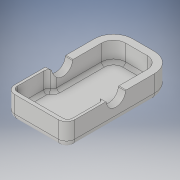
# Autodesk Inventor part: Component 27 (Bracket Cover)
Saved by Autodesk Inventor 2018 (Build 220112000, 112)
## iProperties
Created: 2023-03-30
Part Number: Component 27 (Bracket Cover)
Material: Generic
Document SubType Name: Modeling
Designer: Habib Mohamed
Density: 1 g/cm^3
Appearance: Default
Author: Habib Mohamed
Autodesk Inventor part; units mm, degrees
ref_plane "YZ Plane" through (0, 0, 0) normal (1, 0, 0) x (0, 1, 0)
ref_plane "XZ Plane" through (0, 0, 0) normal (0, 1, 0) x (-1, 0, 0)
ref_plane "XY Plane" through (0, 0, 0) normal (0, 0, 1) x (1, 0, 0)
sketch "Sketch1" plane through (0, 0, 0) normal (0, 1, 0) x (-1, 0, 0)
  line L0 (9, 22.25) -> (-9, 22.25)
  line L1 (-12.5, 18.75) -> (-12.5, -14.25)
  line L2 (-4.5, -22.25) -> (4.5, -22.25)
  line L3 (12.5, -14.25) -> (12.5, 18.75)
  line L4 (12.5, 22.25) -> (-12.5, -22.25) construction
  line L5 (-12.5, 22.25) -> (12.5, -22.25) construction
  line L6 (4.5, -19.25) -> (-4.5, -19.25)
  line L7 (-9.5, -14.25) -> (-9.5, 4.2859)
  line L8 (-11.5, 8.2009) -> (-11.5, 18.75)
  line L9 (-9.5, 20.75) -> (9.5, 20.75)
  line L10 (11.5, 18.75) -> (11.5, 7.75)
  line L11 (9.5, 4.2859) -> (9.5, -14.25)
  arc A0 (4.5, -22.25) -> (12.5, -14.25) centre (4.5, -14.25) ccw
  arc A1 (-12.5, -14.25) -> (-4.5, -22.25) centre (-4.5, -14.25) ccw
  arc A2 (12.5, 18.75) -> (9, 22.25) centre (9, 18.75) ccw
  arc A3 (-9, 22.25) -> (-12.5, 18.75) centre (-9, 18.75) ccw
  arc A4 (4.5, -19.25) -> (9.5, -14.25) centre (4.5, -14.25) ccw
  arc A5 (-9.5, -14.25) -> (-4.5, -19.25) centre (-4.5, -14.25) ccw
  arc A6 (11.5, 18.75) -> (9.5, 20.75) centre (9.5, 18.75) ccw
  arc A7 (-9.5, 20.75) -> (-11.5, 18.75) centre (-9.5, 18.75) ccw
  arc A8 (10.5, 6.0179) -> (11.5, 7.75) centre (9.5, 7.75) ccw
  arc A9 (10.5, 6.0179) -> (9.5, 4.2859) centre (11.5, 4.2859) ccw
  line L12 (0, 0) -> (0, -13.5024) construction
  arc A10 (-11.5, 7.75) -> (-10.5, 6.0179) centre (-9.5, 7.75) ccw
  arc A11 (-9.5, 4.2859) -> (-10.5, 6.0179) centre (-11.5, 4.2859) ccw
  line L13 (-11.5, 7.75) -> (-11.5, 8.2718)
  dimension "d0" = 25
  dimension "d1" = 44.5
  dimension "d2" = 8
  dimension "d3" = 3.5
  dimension "d4" = 5
  dimension "d5" = 2
  dimension "d6" = 3
  dimension "d7" = 1.5
  dimension "d8" = 1
  dimension "d9" = 1
  dimension "d10" = 3
  dimension "d11" = 3
  dimension "d12" = 4
  dimension "d13" = 4
  dimension "d14" = 11
  constraints: 28 end point, 24 point on circle, 19 tangent, 12 centre point, 9 point on line, 4 equal radius, 4 perpendicular, 3 parallel, 3 symmetric about line, 2 horizontal, 2 midpoint, 1 vertical, 2 other
  measures "d0" distance of L4.end L5.end
  measures "d1" distance of L5.end L4.start
  measures "d2" radius of A0
  measures "d3" radius of A2
  measures "d4" radius of A4
  measures "d5" radius of A6
  measures "d6" distance between parallel lines of L2 L6
  measures "d7" distance between parallel lines of L0 L9
  measures "d8" distance between parallel lines of L3 L10
  measures "d9" distance between parallel lines of L1 L8
  measures "d10" distance between parallel lines of L1 L7
  measures "d11" distance between parallel lines of L3 L11
  measures "d12" diameter of A9
  measures "d13" diameter of A8
  measures "d14" vertical distance of L10.start A8.centre
extrude "Extrusion1" add sketch "Sketch1" along normal blind 10 contours A2 L3 A0 L2 A1 L1 A3 L0 | L6 A5 L7 A11 A10 L13 L8 A7 L9 A6 L10 A8 A9 L11 A4
extrude "Extrusion3" cut sketch "Sketch1" against normal blind 8 from surface at 10 contours L6 A5 L7 A11 A10 L13 L8 A7 L9 A6 L10 A8 A9 L11 A4
sketch "Sketch2" plane through (0, 0, 0) normal (1, 0, 0) x (0, 1, 0)
  circle A0 centre (10, 1.75) radius 4
  line L0 (0, -22.25) -> (0, 22.25) construction
  line L1 (0, 22.25) -> (10, 22.25) construction
  line L2 (10, 22.25) -> (10, 20.75) construction
  line L3 (10, 20.75) -> (2, 20.75) construction
  line L4 (2, 20.75) -> (2, -19.25) construction
  line L5 (2, -19.25) -> (10, -19.25) construction
  line L6 (10, -19.25) -> (10, -22.25) construction
  line L7 (10, -22.25) -> (0, -22.25) construction
  point P0 (0, 0)
  dimension "d21" = 8
  dimension "d22" = 24
  dimension "d23" = 10
  constraints: 1 centre point
  measures "d21" diameter of A0
  measures "d22" distance from line of L7 A0.centre
  measures "d23" distance from line of L0 A0.centre
extrude "Extrusion4" cut sketch "Sketch2" along normal mid plane 78.5
fillet "Fillet1" radius 1.25 14 edges at (-9.7679, 2, 5.2859) (-11.2321, 2, 6.75) (-11.5, 2, 13.25) (-10.9142, 2, 20.1642) (0, 2, 20.75) (10.9142, 2, 20.1642) (11.5, 2, 13.25) (11.2321, 2, 6.75) (9.7679, 2, 5.2859) (9.5, 2, -4.9821) (8.0355, 2, -17.7855) (0, 2, -19.25) (-8.0355, 2, -17.7855) (-9.5, 2, -4.9821)
fillet "Fillet2" radius 3 8 edges at (10.1569, 0, -19.9069) (0, 0, -22.25) (-10.1569, 0, -19.9069) (-12.5, 0, 2.25) (-11.4749, 0, 21.2249) (0, 0, 22.25) (11.4749, 0, 21.2249) (12.5, 0, 2.25)
fillet "Fillet3" radius 0.25 4 edges at (-11.3187, 10, 5.75) (-11, 10, -2.25) (11.3187, 10, 5.75) (11, 10, -2.25)
body "Solid1"
